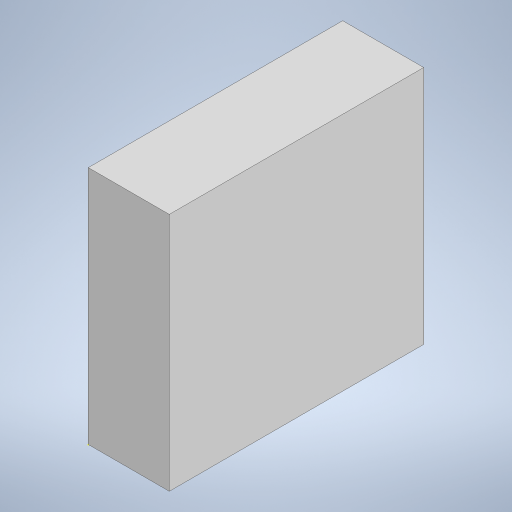
# Autodesk Inventor part: imu_fix
Saved by Autodesk Inventor 2023 (Build 270158000, 158)
## iProperties
Created: 2023-04-06
Part Number: imu_fix
Material: Generic
Document SubType Name: Modeling
Designer: LAB-505
Mass: 20 g
Surface Area: 30.7888 cm^2
Volume: 9.2944 cm^3
Density: 2.15183 g/cm^3
Appearance: Default
Author: LAB-505
Autodesk Inventor part; units mm, degrees
ref_plane "YZ Plane" through (0, 0, 0) normal (1, 0, 0) x (0, 1, 0)
ref_plane "XZ Plane" through (0, 0, 0) normal (0, 1, 0) x (-1, 0, 0)
ref_plane "XY Plane" through (0, 0, 0) normal (0, 0, 1) x (1, 0, 0)
sketch "Sketch1" plane through (0, 0, 0) normal (1, 0, 0) x (0, 1, 0)
  point P0 (0, 0)
sketch "Sketch2" plane through (0, 0, 0) normal (1, 0, 0) x (0, 1, 0)
  line L0 (0, 0) -> (29.6, 0)
  line L1 (29.6, 0) -> (29.6, -31.4)
  line L2 (29.6, -31.4) -> (0, -31.4)
  line L3 (0, -31.4) -> (0, 0)
  dimension "d0" = 29.6
  dimension "d1" = 31.4
  constraints: 8 end point, 2 parallel, 1 horizontal, 1 perpendicular
  measures "d0" distance of L1.end L2.end
  measures "d1" distance of L0.end L1.end
extrude "Extrusion1" add sketch "Sketch2" along normal blind 10
body "Solid1"
